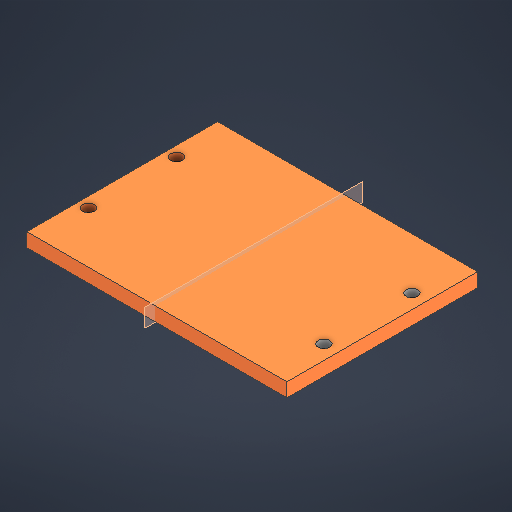
# Autodesk Inventor part: cooling plate
Saved by Autodesk Inventor 2026.2 (Build 302298000, 298)
## iProperties
Created: 2024-12-04
Part Number: cooling plate
Material: Generic
Document SubType Name: Modeling
Designer: cbast
Density: 1 g/cm^3
Appearance: Default
Author: cbast
Autodesk Inventor part; units mm, degrees
ref_plane "YZ Plane" through (0, 0, 0) normal (1, 0, 0) x (0, 1, 0)
ref_plane "XZ Plane" through (0, 0, 0) normal (0, 1, 0) x (-1, 0, 0)
ref_plane "XY Plane" through (0, 0, 0) normal (0, 0, 1) x (1, 0, 0)
sketch "Sketch1" plane through (0, 0, 0) normal (0, 1, 0) x (-1, 0, 0)
  line L0 (-75, 55) -> (75, 55)
  line L1 (75, 55) -> (75, -55)
  line L2 (75, -55) -> (-75, -55)
  line L3 (-75, -55) -> (-75, 55)
  line L4 (-75, 55) -> (75, -55) construction
  line L5 (75, 55) -> (-75, -55) construction
  point P0 (0, 0)
  dimension "d0" = 150
  dimension "d1" = 110
  constraints: 12 end point, 2 midpoint, 2 parallel, 1 horizontal, 1 perpendicular
  measures "d0" distance of L1.end L2.end
  measures "d1" distance of L0.end L1.end
extrude "Extrusion1" add sketch "Sketch1" along normal blind 8
sketch "Sketch9" plane through (0, 8, 0) normal (0, 1, 0) x (1, 0, 0)
  line L0 (-75, 55) -> (-75, -55) construction
  line L1 (-75, -55) -> (75, -55) construction
  line L2 (-62, 57.15) -> (-62, -57.15) construction
  line L3 (75, 55) -> (-75, 55) construction
  line L4 (75, 55) -> (-75, 55) construction
  line L5 (75, -55) -> (75, 55) construction
  line L6 (62, -57.15) -> (62, 57.15) construction
  line L7 (-75, -55) -> (75, -55) construction
  line L8 (-75, -57.15) -> (-62, -57.15) construction
  line L9 (-69.1, 0) -> (-69.1, -25.4) construction
  line L10 (-69.1, 0) -> (-69.1, 25.4) construction
  circle A0 centre (-69.1, 25.4) radius 3.365
  circle A1 centre (-69.1, -25.4) radius 3.365
  point P0 (0, 0)
  point P1 (54, 57.15)
  point P2 (54, -57.15)
  point P3 (-54, -57.15)
  point P4 (-54, 57.15)
  dimension "d36" = 25.4
  dimension "d37" = 25.4
  dimension "d38" = 6.73
  dimension "d39" = 6.73
  constraints: 4 end point, 2 centre point, 2 coincident, 1 parallel, 7 other
  measures "d36" distance of L9.start L9.end
  measures "d37" distance of L9.start L10.end
  measures "d38" diameter of A0
  measures "d39" diameter of A1
extrude "Extrusion9" cut sketch "Sketch9" against normal blind 10
ref_plane "Work Plane2" through (-1.2, 0, 55) normal (1, 0, 0) x (0, 0, -1)
mirror "Mirror2" about plane through (-1.2, 0, 55) normal (1, 0, 0) of "Extrusion9"
body "Solid1"
